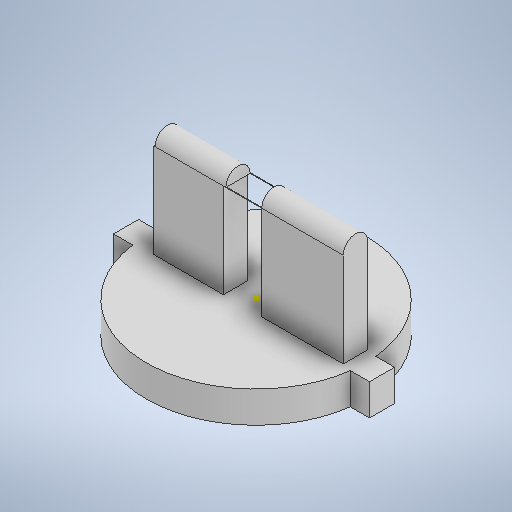
# Autodesk Inventor part: joy part 2
Saved by Autodesk Inventor 2025.2 (Build 292293000, 293)
## iProperties
Created: 2025-03-25
Part Number: joy part 2
Material: Generic
Document SubType Name: Modeling
Designer: avnr2
Density: 1 g/cm^3
Appearance: Default
Author: avnr2
Autodesk Inventor part; units mm, degrees
ref_plane "YZ Plane" through (0, 0, 0) normal (1, 0, 0) x (0, 1, 0)
ref_plane "XZ Plane" through (0, 0, 0) normal (0, 1, 0) x (-1, 0, 0)
ref_plane "XY Plane" through (0, 0, 0) normal (0, 0, 1) x (1, 0, 0)
sketch "Sketch1" plane through (0, 0, 0) normal (0, 1, 0) x (-1, 0, 0)
  line L0 (-34.8245, 0.6257) -> (-40.8245, 0.6257)
  line L1 (-40.8245, 0.6257) -> (-40.8245, 4.6257)
  line L2 (-40.8245, 4.6257) -> (-34.693, 4.6257)
  line L3 (-40.8245, 0.6257) -> (-40.8245, -3.3743)
  line L4 (-40.8245, -3.3743) -> (-34.837, -3.3743)
  line L5 (0, 23.9304) -> (0, -22.2454)
  line L6 (34.8245, 0.6257) -> (40.8245, 0.6257)
  line L7 (40.8245, 0.6257) -> (40.8245, 4.6257)
  line L8 (40.8245, 4.6257) -> (34.693, 4.6257)
  line L9 (40.8245, 0.6257) -> (40.8245, -3.3743)
  line L10 (40.8245, -3.3743) -> (34.837, -3.3743)
  arc A0 (34.693, 4.6257) -> (-34.693, 4.6257) centre (0, 0) ccw
  arc A1 (-34.837, -3.3743) -> (34.837, -3.3743) centre (0, 0) ccw
  point P0 (-34.693, -3.3743)
  point P1 (34.693, -3.3743)
  dimension "d1" = 4
  dimension "d2" = 6
  dimension "d5" = 35
  dimension "d6" = 35
  constraints: 22 end point, 8 symmetric about line, 4 point on circle, 2 centre point, 2 perpendicular, 2 point on line, 1 coincident, 1 horizontal, 1 vertical
  measures "d1" distance of L0.end L1.end
  measures "d2" distance of L0.start L0.end
  measures "d5" radius of A1
  measures "d6" radius of A0
extrude "Extrusion1" add sketch "Sketch1" along normal blind 10
sketch "Sketch2" plane through (0, 10, 0) normal (0, 1, 0) x (1, 0, 0)
  point P0 (0, 0)
sketch "Sketch3" plane through (0, 10, 0) normal (0, 1, 0) x (1, 0, 0)
  point P0 (0, 0)
sketch "Sketch4" plane through (0, 10, 0) normal (0, 1, 0) x (1, 0, 0)
  line L0 (-28.6835, 3.8877) -> (-6.4953, 3.8877)
  line L1 (-6.4953, 3.8877) -> (-6.4953, -3.8877)
  line L2 (-6.4953, -3.8877) -> (-28.6835, -3.8877)
  line L3 (-28.6835, -3.8877) -> (-28.6835, 3.8877)
  line L4 (-28.6835, 3.8877) -> (-6.4953, -3.8877) construction
  line L5 (-6.4953, 3.8877) -> (-28.6835, -3.8877) construction
  line L6 (5.7367, 3.8877) -> (31.7178, 3.8877)
  line L7 (31.7178, 3.8877) -> (31.7178, -3.8877)
  line L8 (31.7178, -3.8877) -> (5.7367, -3.8877)
  line L9 (5.7367, -3.8877) -> (5.7367, 3.8877)
  line L10 (5.7367, 3.8877) -> (31.7178, -3.8877) construction
  line L11 (31.7178, 3.8877) -> (5.7367, -3.8877) construction
  point P0 (0, 0)
  point P1 (-17.5894, 0)
  point P2 (18.7272, 0)
  constraints: 24 end point, 4 midpoint, 4 parallel, 2 horizontal, 2 perpendicular, 1 point on line
extrude "Extrusion2" add sketch "Sketch4" along normal blind 30
sketch "Sketch5" plane through (31.7178, 10, 3.8877) normal (1, 0, 0) x (0, 0, -1)
  line L0 (7.7754, 30) -> (0, 30) projected
  arc A0 (7.7754, 30) -> (0, 30) centre (3.8877, 30.1095) ccw
  point P0 (3.8877, -10)
  constraints: 2 point on circle, 1 centre point
extrude "Extrusion3" add sketch "Sketch5" against normal blind 60
sketch "Sketch6" plane through (0, 10, 0) normal (0, 1, 0) x (1, 0, 0)
  line L0 (5.7367, -3.8877) -> (5.7367, 3.8877) projected
  line L1 (-5.7367, 3.8877) -> (5.7367, 3.8877)
  line L2 (5.7367, 3.8877) -> (5.7367, -3.8877)
  line L3 (5.7367, -3.8877) -> (-5.7367, -3.8877)
  line L4 (-5.7367, -3.8877) -> (-5.7367, 3.8877)
  line L5 (-5.7367, 3.8877) -> (5.7367, -3.8877) construction
  line L6 (5.7367, 3.8877) -> (-5.7367, -3.8877) construction
  point P0 (0, 0)
  constraints: 12 end point, 2 midpoint, 2 parallel, 1 horizontal, 1 perpendicular
extrude "Extrusion4" cut sketch "Sketch6" along normal blind 60
body "Solid1"
